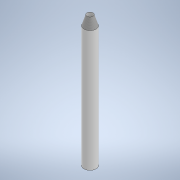
# Autodesk Inventor part: rev pen
Saved by Autodesk Inventor 2022 (Build 260153000, 153)
## iProperties
Created: 2021-07-09
Part Number: rev pen
Material: Generic
Document SubType Name: Modeling
Designer: User
Density: 1 g/cm^3
Appearance: Default
Author: User
Autodesk Inventor part; units mm, degrees
ref_plane "YZ Plane" through (0, 0, 0) normal (1, 0, 0) x (0, 1, 0)
ref_plane "XZ Plane" through (0, 0, 0) normal (0, 1, 0) x (-1, 0, 0)
ref_plane "XY Plane" through (0, 0, 0) normal (0, 0, 1) x (1, 0, 0)
sketch "Sketch1" plane through (0, 0, 0) normal (0, 0, 1) x (1, 0, 0)
  line L0 (-4.4815, 191.0665) -> (-4.4815, -8.9335)
  line L1 (-4.4815, -8.9335) -> (-14.4815, -8.9335)
  line L2 (-14.4815, -8.9335) -> (-14.4815, 191.0665)
  line L3 (-14.4815, 191.0665) -> (-9.4815, 206.8311)
  line L4 (-9.4815, 206.8311) -> (-4.4815, 191.0665)
  point P0 (0, 0)
  dimension "d0" = 10
  dimension "d1" = 200
  constraints: 10 end point, 1 parallel
  measures "d0" distance of L0.end L1.end
  measures "d1" distance of L0.start L0.end
revolve "Revolution1" add sketch "Sketch1" angle 360 about axis through (-4.4815, 191.0665, 0) along (0, -1, 0)
thread "Thread1" size "R 1/16" standard "ISO Taper" full length
body "Solid1"
